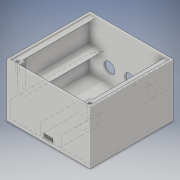
# Autodesk Inventor part: teensy_box
Saved by Autodesk Inventor 2017 (Build 210142000, 142)
## iProperties
Created: 2016-09-19
Part Number: teensy_box
Material: Generic
Document SubType Name: Modeling
Designer: corvera
Density: 1 g/cm^3
Appearance: Default
Author: corvera
Autodesk Inventor part; units mm, degrees
ref_plane "YZ Plane" through (0, 0, 0) normal (1, 0, 0) x (0, 1, 0)
ref_plane "XZ Plane" through (0, 0, 0) normal (0, 1, 0) x (-1, 0, 0)
ref_plane "XY Plane" through (0, 0, 0) normal (0, 0, 1) x (1, 0, 0)
sketch "Sketch1" plane through (0, 0, 0) normal (0, 1, 0) x (-1, 0, 0)
  line L0 (40.5, 40.5) -> (-40.5, 40.5)
  line L1 (-40.5, 40.5) -> (-40.5, -40.5)
  line L2 (-40.5, -40.5) -> (40.5, -40.5)
  line L3 (40.5, -40.5) -> (40.5, 40.5)
  line L4 (40.5, 40.5) -> (-40.5, -40.5) construction
  line L5 (-40.5, 40.5) -> (40.5, -40.5) construction
  point P0 (0, 0)
  dimension "box_width" = 81
  dimension "box_height" = 81
  constraints: 12 end point, 2 midpoint, 2 parallel, 1 horizontal, 1 perpendicular
  measures "box_width" distance of L1.end L2.end
  measures "box_height" distance of L0.end L1.end
extrude "Base" add sketch "Sketch1" against normal blind 1.5
sketch "Sketch2" plane through (0, 0, 0) normal (0, 1, 0) x (-1, 0, 0)
  line L0 (40.5, -40.5) -> (-40.5, -40.5) projected
  line L1 (40.5, 40.5) -> (-40.5, 40.5)
  line L2 (-40.5, 40.5) -> (-40.5, -40.5)
  line L3 (-40.5, -40.5) -> (40.5, -40.5)
  line L4 (40.5, -40.5) -> (40.5, 40.5)
  line L5 (40.5, 40.5) -> (-40.5, -40.5) construction
  line L6 (-40.5, 40.5) -> (40.5, -40.5) construction
  line L7 (38.5, 38.5) -> (-38.5, 38.5)
  line L8 (-38.5, 38.5) -> (-38.5, -38.5)
  line L9 (-38.5, -38.5) -> (38.5, -38.5)
  line L10 (38.5, -38.5) -> (38.5, 38.5)
  line L11 (38.5, 38.5) -> (-38.5, -38.5) construction
  line L12 (-38.5, 38.5) -> (38.5, -38.5) construction
  point P0 (0, 0)
  dimension "wall_thickness" = 2
  constraints: 24 end point, 4 midpoint, 4 parallel, 2 horizontal, 2 perpendicular, 1 point on line
  measures "wall_thickness" distance between parallel lines of L0 L9
extrude "Wall" add sketch "Sketch2" along normal blind 50
sketch "Sketch3" plane through (0, 0, 0) normal (0, 1, 0) x (-1, 0, 0)
  line L0 (-9.75, 39.5) -> (9.75, 39.5)
  line L1 (9.75, 39.5) -> (9.75, 1.7)
  line L2 (9.75, 1.7) -> (-9.75, 1.7)
  line L3 (-9.75, 1.7) -> (-9.75, 39.5)
  line L4 (-9.75, 39.5) -> (9.75, 1.7) construction
  line L5 (9.75, 39.5) -> (-9.75, 1.7) construction
  line L6 (0, 20.6) -> (0, 0) construction
  line L7 (10.75, 40.5) -> (-10.75, 40.5)
  line L8 (-10.75, 40.5) -> (-10.75, 0.7)
  line L9 (-10.75, 0.7) -> (10.75, 0.7)
  line L10 (10.75, 0.7) -> (10.75, 40.5)
  line L11 (10.75, 40.5) -> (-10.75, 0.7) construction
  line L12 (-10.75, 40.5) -> (10.75, 0.7) construction
  line L13 (40.5, 40.5) -> (-40.5, 40.5) projected
  point P0 (0, 40.5)
  dimension "d7" = 37.8
  dimension "d8" = 19.5
  dimension "d9" = 1
  dimension "d10" = 1
  constraints: 26 end point, 6 midpoint, 4 parallel, 2 horizontal, 2 perpendicular, 1 vertical
  measures "d7" distance of L0.end L1.end
  measures "d8" distance of L1.end L2.end
  measures "d9" distance between parallel lines of L2 L9
  measures "d10" distance between parallel lines of L3 L8
extrude "Teensy Wall" add sketch "Sketch3" along normal blind 10
sketch "Sketch4" plane through (40.5, -1.5, -40.5) normal (0, 0, -1) x (-1, 0, 0)
  line L0 (79, 51.5) -> (2, 51.5) construction
  line L1 (2, 51.5) -> (79, 51.5) construction
  line L2 (40.5, 51.5) -> (40.5, 15) construction
  line L3 (40.5, 15) -> (20.5, 15) construction
  circle A0 centre (20.5, 15) radius 5.5
  line L4 (40.5, 15) -> (40.5, 0) construction
  line L5 (81, 0) -> (0, 0) construction
  circle A1 centre (40.5, 15) radius 5.5
  circle A2 centre (60.5, 15) radius 5.5
  dimension "d21" = 11
  dimension "d23" = 20
  dimension "d59" = 20
  constraints: 6 end point, 3 centre point, 2 midpoint, 1 coincident, 1 horizontal, 1 perpendicular, 1 vertical, 4 other
  measures "d21" diameter of A0
  measures "d23" distance of L2.end L3.end
  measures "d59" distance of A0.centre A1.centre
extrude "BNC Holes" cut sketch "Sketch4" against normal up to surface (2 mm away)
sketch "Sketch7" plane through (-38.5, 0, -38.5) normal (0, 0, 1) x (1, 0, 0)
  line L0 (79, 50) -> (-2, 50) projected
  line L1 (-2, -1.5) -> (-2, 50) projected
  line L2 (-2, 50) -> (-2, 25) construction
  line L3 (-2, 25) -> (13, 25)
  line L4 (13, 25) -> (-2, 15)
  line L5 (-2, 15) -> (-2, 25)
  line L6 (38.5, 50) -> (38.5, 0) construction
  line L7 (79, -1.5) -> (79, 50)
  line L8 (79, 50) -> (79, 25) construction
  line L9 (79, 25) -> (64, 25)
  line L10 (64, 25) -> (79, 15)
  line L11 (79, 15) -> (79, 25)
  point P0 (-2, 30)
  dimension "d32" = 25
  dimension "d33" = 10
  dimension "d34" = 15
  constraints: 20 end point, 4 symmetric about line, 3 vertical, 1 horizontal, 1 midpoint, 1 point on line
  measures "d32" distance of L0.end L2.end
  measures "d33" distance of L4.end L2.end
  measures "d34" distance of L2.end L3.end
extrude "Battery Support" add sketch "Sketch7" along normal up to next
sketch "Sketch8" plane through (-40.5, -1.5, 40.5) normal (0, 0, 1) x (1, 0, 0)
  line L0 (79, 51.5) -> (2, 51.5) construction
  line L1 (40.5, 51.5) -> (40.5, 1.5) construction
  line L2 (36, 3.5) -> (45, 3.5)
  line L3 (45, 3.5) -> (45, 7.5)
  line L4 (45, 7.5) -> (36, 7.5)
  line L5 (36, 7.5) -> (36, 3.5)
  line L6 (36, 3.5) -> (45, 7.5) construction
  line L7 (45, 3.5) -> (36, 7.5) construction
  point P0 (40.5, 5.5)
  dimension "d36" = 9
  dimension "d37" = 4
  dimension "d38" = 2
  constraints: 14 end point, 3 midpoint, 2 parallel, 1 horizontal, 1 perpendicular, 1 point on line, 1 vertical
  measures "d36" distance of L2.start L2.end
  measures "d37" distance of L2.end L3.end
  measures "d38" distance from line of L2 L1.end
extrude "USB Hole" cut sketch "Sketch8" against normal up to next
sketch "Sketch9" plane through (-38.5, 25, -38.5) normal (0, 1, 0) x (1, 0, 0)
  line L0 (0, 0) -> (77, 0) projected
  line L1 (64, 0) -> (64, -77) projected
  line L2 (49.25, -77) -> (77, -77) projected
  line L3 (77, 0) -> (77, -77) projected
  line L4 (85.7069, 0) -> (84.513, 0)
  line L5 (77, -77) -> (70, -77)
  line L6 (70, -77) -> (70, -70)
  line L7 (70, -70) -> (77, -70)
  line L8 (77, -70) -> (77, -77)
  line L9 (77, 0) -> (0, 0) projected
  line L10 (0, -77) -> (5.9059, -77)
  line L11 (0, -77) -> (5.9059, -77)
  line L12 (0, -77) -> (7, -77)
  line L13 (7, -77) -> (7, -70)
  line L14 (7, -70) -> (0, -70)
  line L15 (0, -70) -> (0, -77)
  line L16 (77, -77) -> (0, -77) projected
  line L17 (0, -77) -> (0, 0) projected
  dimension "d66" = 7
  constraints: 22 end point, 8 equal length, 5 collinear, 2 perpendicular, 1 horizontal
  measures "d66" distance of L6.end L7.end
extrude "Plate Support" add sketch "Sketch9" along normal blind 23.5 contours L14 L13 L12 L10 L15 | L3 L2 L6 L7
sketch "Sketch15" plane through (-38.5, 0, -38.5) normal (0, 0, 1) x (1, 0, 0)
  line L0 (-2, 48.5) -> (-2, 41.5)
  line L1 (-2, 41.5) -> (5, 48.5)
  line L2 (5, 48.5) -> (-2, 48.5)
  line L3 (-2, -1.5) -> (-2, 50) projected
  line L4 (79, 50) -> (-2, 50) projected
  line L5 (38.5, 50) -> (38.5, -1.5)
  line L6 (-2, -1.5) -> (79, -1.5) projected
  line L7 (79, 48.5) -> (79, 41.5)
  line L8 (79, 41.5) -> (72, 48.5)
  line L9 (72, 48.5) -> (79, 48.5)
  point P0 (38.5, 0)
  dimension "d70" = 7
  dimension "d71" = 1.5
  constraints: 14 end point, 3 symmetric about line, 2 midpoint, 1 collinear, 1 horizontal, 1 perpendicular, 1 vertical
  measures "d70" distance of L1.end L0.start
  measures "d71" distance between parallel lines of L2 L4
extrude "Extrusion12" add sketch "Sketch15" along normal up to surface (79 mm away) contours L2 L1 L0 | L7 L8 L9
sketch "Sketch14" plane through (-38.5, 48.5, -38.5) normal (0, 1, 0) x (1, 0, 0)
  circle A0 centre (3.5, -73.5) radius 1.45
  line L0 (7, -70) -> (7, -77) construction
  line L1 (3.5, -73.5) -> (7, -70) construction
  line L2 (3.5, -73.5) -> (7, -77) construction
  line L3 (77, -77) -> (0, -77) construction
  line L4 (0, -77) -> (3.5, -73.5) construction
  circle A1 centre (73.5, -73.5) radius 1.45
  line L5 (70, -77) -> (70, -70) construction
  line L6 (70, -70) -> (73.5, -73.5) construction
  line L7 (70, -70) -> (77, -70) construction
  line L8 (73.5, -73.5) -> (77, -70) construction
  line L9 (73.5, -73.5) -> (70, -77) construction
  point P0 (38.5, -38.5)
  dimension "d67" = 2.9
  constraints: 12 end point, 4 perpendicular, 2 centre point, 1 equal radius
  measures "d67" diameter of A0
extrude "Extrusion11" cut sketch "Sketch14" against normal blind 10
body "Solid1"
